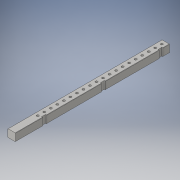
# Autodesk Inventor part: Post
Saved by Autodesk Inventor 2016 (Build 200138000, 138)
## iProperties
Created: 2016-07-05
Part Number: Post
Material: Generic
Document SubType Name: Modeling
Designer: kurti
Density: 1 g/cm^3
Appearance: Default
Author: kurti
Autodesk Inventor part; units mm, degrees
ref_plane "YZ Plane" through (0, 0, 0) normal (1, 0, 0) x (0, 1, 0)
ref_plane "XZ Plane" through (0, 0, 0) normal (0, 1, 0) x (-1, 0, 0)
ref_plane "XY Plane" through (0, 0, 0) normal (0, 0, 1) x (1, 0, 0)
sketch "Sketch1" plane through (0, 0, 0) normal (0, 0, 1) x (1, 0, 0)
  line L0 (-44.45, -44.45) -> (44.45, -44.45)
  line L1 (44.45, -44.45) -> (44.45, 44.45)
  line L2 (44.45, 44.45) -> (-44.45, 44.45)
  line L3 (-44.45, 44.45) -> (-44.45, -44.45)
  line L4 (-44.45, -44.45) -> (44.45, 44.45) construction
  line L5 (44.45, -44.45) -> (-44.45, 44.45) construction
  point P0 (0, 0)
  dimension "d0" = 88.9
  dimension "d1" = 88.9
  constraints: 12 end point, 2 midpoint, 2 parallel, 1 horizontal, 1 perpendicular
  measures "d0" distance of L2.end L1.end
  measures "d1" distance of L1.end L0.end
extrude "4x4 Stock" add sketch "Sketch1" along normal blind 1828.8
sketch "Sketch2" plane through (-44.45, 44.45, 0) normal (0, 1, 0) x (1, 0, 0)
  line L0 (0, -1828.8) -> (88.9, -1828.8) construction
  line L1 (88.9, -1828.8) -> (88.9, -1511.3) construction
  line L2 (88.9, 0) -> (88.9, -1828.8) construction
  line L3 (88.9, -1511.3) -> (76.2, -1511.3)
  line L4 (88.9, -1511.3) -> (101.6, -1511.3) construction
  line L5 (76.2, -1511.3) -> (76.2, -1466.85)
  line L6 (76.2, -1466.85) -> (88.9, -1466.85)
  line L7 (88.9, -1828.8) -> (88.9, -825.5) construction
  line L8 (88.9, -825.5) -> (76.2, -825.5)
  line L9 (76.2, -825.5) -> (76.2, -781.05)
  line L10 (76.2, -781.05) -> (88.9, -781.05)
  line L11 (88.9, -1828.8) -> (88.9, -152.4) construction
  line L12 (88.9, -152.4) -> (76.2, -152.4)
  line L13 (76.2, -152.4) -> (76.2, -107.95)
  line L14 (76.2, -107.95) -> (88.9, -107.95)
  line L15 (88.9, -825.5) -> (88.9, -781.05)
  line L16 (88.9, -152.4) -> (88.9, -107.95)
  line L17 (88.9, -1511.3) -> (88.9, -1466.85)
  point P0 (44.45, 0)
  dimension "d4" = 317.5
  dimension "d5" = 12.7
  dimension "d6" = 180
  dimension "d7" = 44.45
  dimension "d8" = 1003.3
  dimension "d9" = 12.7
  dimension "d10" = 44.45
  dimension "d11" = 1676.4
  dimension "d12" = 12.7
  dimension "d13" = 44.45
  constraints: 32 end point, 8 point on line, 6 perpendicular, 3 collinear, 2 horizontal, 1 vertical
  measures "d4" distance of L0.end L1.end
  measures "d5" distance of L1.end L3.end
  measures "d6" angle of L3 L4
  measures "d7" distance of L3.end L5.end
  measures "d8" distance of L0.end L7.end
  measures "d9" distance of L7.end L8.end
  measures "d10" distance of L8.end L9.end
  measures "d11" distance of L0.end L11.end
  measures "d12" distance of L11.end L12.end
  measures "d13" distance of L12.end L13.end
extrude "Center Support Slots" cut sketch "Sketch2" against normal blind 101.6
sketch "Sketch3" plane through (-44.45, 44.45, 0) normal (0, 1, 0) x (1, 0, 0)
  line L0 (88.9, -1828.8) -> (0, -1828.8) construction
  line L1 (44.45, -1828.8) -> (44.45, -1524) construction
  line L2 (44.45, -1524) -> (44.45, -1447.8) construction
  line L3 (44.45, -1447.8) -> (44.45, -1371.6) construction
  line L4 (44.45, -1371.6) -> (44.45, -1295.4) construction
  line L5 (44.45, -1295.4) -> (44.45, -1219.2) construction
  line L6 (44.45, -1219.2) -> (44.45, -1143) construction
  line L7 (44.45, -1143) -> (44.45, -1066.8) construction
  line L8 (44.45, -1066.8) -> (44.45, -990.6) construction
  line L9 (44.45, -990.6) -> (44.45, -914.4) construction
  line L10 (44.45, -914.4) -> (44.45, -838.2) construction
  line L11 (44.45, -838.2) -> (44.45, -762) construction
  line L12 (44.45, -762) -> (44.45, -685.8) construction
  line L13 (44.45, -685.8) -> (44.45, -609.6) construction
  line L14 (44.45, -609.6) -> (44.45, -533.4) construction
  line L15 (44.45, -533.4) -> (44.45, -457.2) construction
  line L16 (44.45, -457.2) -> (44.45, -381) construction
  line L17 (44.45, -381) -> (44.45, -304.8) construction
  line L18 (44.45, -304.8) -> (44.45, -228.6) construction
  line L19 (44.45, -228.6) -> (44.45, -152.4) construction
  line L20 (44.45, -152.4) -> (44.45, -76.2) construction
  circle A0 centre (44.45, -1524) radius 12.7
  circle A1 centre (44.45, -1447.8) radius 12.7
  circle A2 centre (44.45, -1371.6) radius 12.7
  circle A3 centre (44.45, -1295.4) radius 12.7
  circle A4 centre (44.45, -1219.2) radius 12.7
  circle A5 centre (44.45, -1143) radius 12.7
  circle A6 centre (44.45, -1066.8) radius 12.7
  circle A7 centre (44.45, -990.6) radius 12.7
  circle A8 centre (44.45, -914.4) radius 12.7
  circle A9 centre (44.45, -838.2) radius 12.7
  circle A10 centre (44.45, -762) radius 12.7
  circle A11 centre (44.45, -685.8) radius 12.7
  circle A12 centre (44.45, -609.6) radius 12.7
  circle A13 centre (44.45, -533.4) radius 12.7
  circle A14 centre (44.45, -457.2) radius 12.7
  circle A15 centre (44.45, -381) radius 12.7
  circle A16 centre (44.45, -304.8) radius 12.7
  circle A17 centre (44.45, -228.6) radius 12.7
  circle A18 centre (44.45, -152.4) radius 12.7
  circle A19 centre (44.45, -76.2) radius 12.7
  point P0 (44.45, 0)
  dimension "d16" = 304.8
  dimension "d17" = 76.2
  dimension "d18" = 76.2
  dimension "d19" = 76.2
  dimension "d20" = 76.2
  dimension "d21" = 76.2
  dimension "d22" = 76.2
  dimension "d23" = 76.2
  dimension "d24" = 76.2
  dimension "d25" = 76.2
  dimension "d26" = 76.2
  dimension "d27" = 76.2
  dimension "d28" = 76.2
  dimension "d29" = 76.2
  dimension "d30" = 76.2
  dimension "d31" = 76.2
  dimension "d32" = 76.2
  dimension "d33" = 76.2
  dimension "d34" = 76.2
  dimension "d35" = 76.2
  dimension "d36" = 25.4
  dimension "d37" = 25.4
  dimension "d38" = 25.4
  dimension "d39" = 25.4
  dimension "d40" = 25.4
  dimension "d41" = 25.4
  dimension "d42" = 25.4
  dimension "d43" = 25.4
  dimension "d44" = 25.4
  dimension "d45" = 25.4
  dimension "d46" = 25.4
  dimension "d47" = 25.4
  dimension "d48" = 25.4
  dimension "d49" = 25.4
  dimension "d50" = 25.4
  dimension "d51" = 25.4
  dimension "d52" = 25.4
  dimension "d53" = 25.4
  dimension "d54" = 25.4
  dimension "d55" = 25.4
  constraints: 40 end point, 20 centre point, 20 coincident, 19 point on line, 1 midpoint, 1 vertical
  measures "d16" distance of L1.start L1.end
  measures "d17" distance of L1.end L2.end
  measures "d18" distance of L2.end L3.end
  measures "d19" distance of L3.end L4.end
  measures "d20" distance of L4.end L5.end
  measures "d21" distance of L5.end L6.end
  measures "d22" distance of L6.end L7.end
  measures "d23" distance of L7.end L8.end
  measures "d24" distance of L8.end L9.end
  measures "d25" distance of L9.end L10.end
  measures "d26" distance of L10.end L11.end
  measures "d27" distance of L11.end L12.end
  measures "d28" distance of L12.end L13.end
  measures "d29" distance of L13.end L14.end
  measures "d30" distance of L14.end L15.end
  measures "d31" distance of L15.end L16.end
  measures "d32" distance of L16.end L17.end
  measures "d33" distance of L17.end L18.end
  measures "d34" distance of L18.end L19.end
  measures "d35" distance of L19.end L20.end
  measures "d36" diameter of A0
  measures "d37" diameter of A1
  measures "d38" diameter of A2
  measures "d39" diameter of A3
  measures "d40" diameter of A4
  measures "d41" diameter of A5
  measures "d42" diameter of A6
  measures "d43" diameter of A7
  measures "d44" diameter of A8
  measures "d45" diameter of A9
  measures "d46" diameter of A10
  measures "d47" diameter of A11
  measures "d48" diameter of A12
  measures "d49" diameter of A13
  measures "d50" diameter of A14
  measures "d51" diameter of A15
  measures "d52" diameter of A16
  measures "d53" diameter of A17
  measures "d54" diameter of A18
  measures "d55" diameter of A19
extrude "Extrusion3" cut sketch "Sketch3" against normal blind 101.6
chamfer "Chamfer1" distance 31.75 angle 45 4 edges at (0, 44.45, 0) (-44.45, 0, 0) (0, -44.45, 0) (44.45, 0, 0)
fillet "Fillet1" radius 3.175 10 edges at (-44.45, -44.45, 930.275) (-44.45, 44.45, 930.275) (44.45, -44.45, 1670.05) (44.45, -44.45, 1146.175) (44.45, -44.45, 466.725) (44.45, -44.45, 69.85) (44.45, 44.45, 69.85) (44.45, 44.45, 466.725) (44.45, 44.45, 1146.175) (44.45, 44.45, 1670.05)
body "Solid1"
